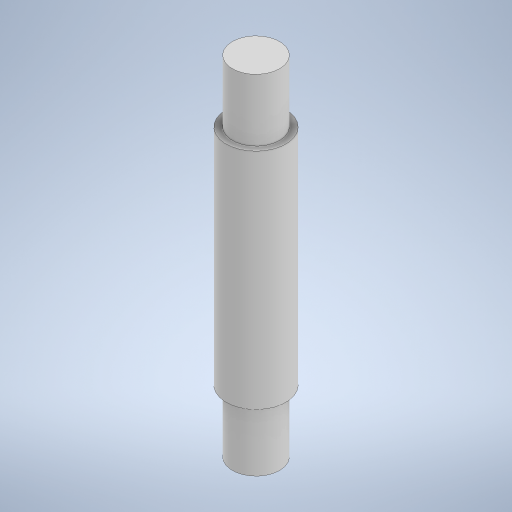
# Autodesk Inventor part: Pieza7
Saved by Autodesk Inventor 2024.3 (Build 283343000, 343)
## iProperties
Created: 2025-02-01
Part Number: Pieza7
Material: Genérico
Document SubType Name: Modeling
Designer: Jorge
Density: 1 g/cm^3
Appearance: Valor por defecto
Author: Jorge
Autodesk Inventor part; units mm, degrees
ref_plane "YZ Plane" through (0, 0, 0) normal (1, 0, 0) x (0, 1, 0)
ref_plane "XY Plane" through (0, 0, 0) normal (0, 0, 1) x (1, 0, 0)
sketch "Boceto1" plane through (0, 0, 0) normal (1, 0, 0) x (0, 1, 0)
  line L0 (0, 0) -> (18, 0)
  line L1 (0, 0) -> (0, -4.8)
  line L2 (18, 0) -> (23, 0)
  line L3 (18, 0) -> (18, -3.8)
  line L4 (0, 0) -> (-5, 0)
  line L5 (-5, 0) -> (-5, 3.8)
  dimension "d0" = 18
  dimension "d1" = 4.8
  dimension "d2" = 5
  dimension "d4" = 3.8
  dimension "d5" = 5
  dimension "d6" = 3.8
  constraints: 12 end point, 3 horizontal, 2 vertical, 1 perpendicular
  measures "d0" distance of L0.start L0.end
  measures "d1" distance of L0.start L1.end
  measures "d2" distance of L0.end L2.end
  measures "d4" distance of L0.end L3.end
  measures "d5" distance of L0.start L4.end
  measures "d6" distance of L4.end L5.end
sketch "Boceto4" plane through (0, 0, 0) normal (0, 1, 0) x (-1, 0, 0)
  circle A0 centre (0, 0) radius 2.4
  dimension "d10" = 4.8
  constraints: 1 centre point, 1 coincident
  measures "d10" diameter of A0
sweep "Barrido1" add profiles "Boceto4" path "Boceto1" path curves L0
ref_plane "Plano de trabajo1" through (0, 9, 0) normal (0, 1, 0) x (-1, 0, 0)
sketch "Boceto5" plane through (0, 9, 0) normal (0, 1, 0) x (-1, 0, 0)
  circle A0 centre (0, 0) radius 1.9
  dimension "d14" = 3.8
  constraints: 1 centre point, 1 coincident
  measures "d14" diameter of A0
extrude "Extrusión1" add sketch "Boceto5" along normal mid plane 28
